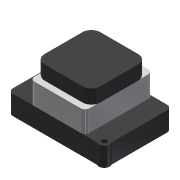
# Autodesk Inventor part: Talon Controller
Saved by Autodesk Inventor 2013 (Build 170138000, 138)
## iProperties
Created: 2013-12-22
Part Number: Talon Controller
Material: Nylon 6/6
Document SubType Name: Modeling
Designer: Nemo
Density: 1.00848 g/cm^3
Mass: 90.7185 g
Surface Area: 210.799 cm^2
Volume: 89.9557 cm^3
Author: Nemo
Autodesk Inventor part; units mm, degrees
ref_plane "YZ Plane" through (0, 0, 0) normal (1, 0, 0) x (0, 1, 0)
ref_plane "XZ Plane" through (0, 0, 0) normal (0, 1, 0) x (-1, 0, 0)
ref_plane "XY Plane" through (0, 0, 0) normal (0, 0, 1) x (1, 0, 0)
sketch "Sketch2" plane through (0, 0, 0) normal (0, 1, 0) x (-1, 0, 0)
  line L0 (-3.3777, 3.3777) -> (-3.3777, 43.0061)
  ellipse E0 centre (0.001, 3.3787) end of major axis (-2.3884, 0.9892) minor radius 3.3782 (-3.3777, 3.3777) -> (0, 0) ccw
  line L1 (59.9484, 0) -> (0, 0)
  ellipse E1 centre (59.9793, -0.3859) end of major axis (60.4086, -0.4945) minor radius 0.3819 (60.193, -0.0627) -> (59.9484, 0) ccw
  arc A0 (60.193, -0.0627) -> (65.3667, 5.111) centre (62.0273, 3.2766) ccw
  arc A1 (65.3039, 5.3555) -> (65.3667, 5.111) centre (65.8118, 5.3555) ccw
  line L2 (65.3039, 44.9839) -> (65.3039, 5.3555)
  ellipse E2 centre (61.9252, 44.9829) end of major axis (59.5357, 42.5934) minor radius 3.3782 (65.3039, 44.9839) -> (61.9262, 48.3616) ccw
  line L3 (1.9778, 48.3616) -> (61.9262, 48.3616)
  arc A2 (1.7333, 48.4243) -> (1.9778, 48.3616) centre (1.9778, 48.8695) ccw
  arc A3 (1.7333, 48.4243) -> (-3.4404, 43.2506) centre (-0.1011, 45.085) ccw
  arc A4 (-3.3777, 43.0061) -> (-3.4404, 43.2506) centre (-3.8856, 43.0061) ccw
  arc A5 (-0.0268, 47.0408) -> (-2.0588, 45.0088) centre (-0.0268, 45.0088) ccw
  line L4 (59.9191, 47.0408) -> (-0.0268, 47.0408) construction
  arc A6 (63.9831, 42.9768) -> (59.9191, 47.0408) centre (59.9191, 42.9768) ccw construction
  line L5 (63.9831, 3.3528) -> (63.9831, 42.9768) construction
  arc A7 (61.9511, 1.3208) -> (63.9831, 3.3528) centre (61.9511, 3.3528) ccw
  line L6 (2.0052, 1.3208) -> (61.9511, 1.3208) construction
  arc A8 (-2.0588, 5.3848) -> (2.0052, 1.3208) centre (2.0052, 5.3848) ccw construction
  line L7 (-2.0588, 45.0088) -> (-2.0588, 5.3848) construction
  circle A9 centre (-0.1011, 45.085) radius 1.905
  circle A10 centre (62.0273, 3.2766) radius 1.905
  constraints: 18 point on circle, 16 end point, 11 centre point, 12 other
extrude "Extrusion1" add sketch "Sketch2" along normal blind 13.8176
sketch "Sketch3" plane through (0, 13.8176, 0) normal (0, 1, 0) x (1, 0, 0)
  line L0 (0, 0) -> (-59.9484, 0) construction
  line L1 (-61.9262, -48.3616) -> (-1.9778, -48.3616) construction
  line L2 (-49.6211, 0) -> (-10.3273, 0)
  line L3 (-10.3273, 0) -> (-10.3273, -48.3616)
  line L4 (-10.3273, -48.3616) -> (-49.6211, -48.3616)
  line L5 (-49.6211, -48.3616) -> (-49.6211, 0)
  point P0 (-29.9742, 0)
  dimension "d2" = 39.2938
  constraints: 8 end point, 2 midpoint, 2 parallel, 2 point on line, 1 horizontal, 1 perpendicular
  measures "d2" distance between parallel lines of L3 L5
extrude "Extrusion2" add sketch "Sketch3" along normal blind 15.24 separate body
fillet "Fillet1" radius 3.175 4 edges at (-49.6211, 21.4376, 0) (-10.3273, 21.4376, 0) (-10.3273, 21.4376, 48.3616) (-49.6211, 21.4376, 48.3616)
sketch "Sketch4" plane through (0, 29.0576, 0) normal (0, 1, 0) x (1, 0, 0)
  line L0 (-13.5023, 0) -> (-46.4461, 0) construction
  line L1 (-49.6211, -3.175) -> (-49.6211, -45.1866) construction
  line L2 (-49.9132, -4.2418) -> (-10.0352, -4.2418)
  line L3 (-10.0352, -4.2418) -> (-10.0352, -44.1198)
  line L4 (-10.0352, -44.1198) -> (-49.9132, -44.1198)
  line L5 (-49.9132, -44.1198) -> (-49.9132, -4.2418)
  point P0 (0, 0)
  point P1 (-29.9742, -4.2418)
  point P2 (-29.9742, 0)
  point P3 (-49.9132, -24.1808)
  point P4 (-49.6211, -24.1808)
  dimension "d7" = 39.878
  dimension "d8" = 39.878
  constraints: 8 end point, 4 midpoint, 2 parallel, 1 horizontal, 1 horizontal alignment, 1 perpendicular, 1 vertical alignment
  measures "d7" distance of L3.end L4.end
  measures "d8" distance of L2.end L3.end
extrude "Extrusion3" add sketch "Sketch4" along normal blind 10 separate body
fillet "Fillet2" radius 6.35 4 edges at (-49.9132, 34.0576, 44.1198) (-10.0352, 34.0576, 44.1198) (-10.0352, 34.0576, 4.2418) (-49.9132, 34.0576, 4.2418)
body "Solid1"
body "Solid2"
body "Solid3"
